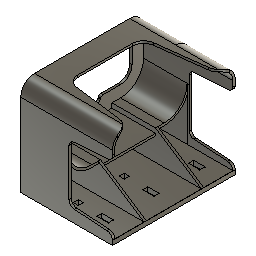
brother_e550w_holder (Autodesk Fusion 360 design; units mm, degrees)
Autodesk Fusion 360 part; units mm, degrees
sketch "Sketch1" plane through (0, 0, 0) normal (1, 0, 0) x (0, 1, 0)
  line L0 (103, 20) -> (103, 42)
  line L1 (93, 52) -> (10, 52)
  line L2 (0, 42) -> (0, 20)
  arc A0 (0, 20) -> (20, 0) centre (20, 20) ccw
  arc A1 (83, 0) -> (103, 20) centre (83, 20) ccw
  arc A2 (10, 52) -> (0, 42) centre (10, 42) ccw
  arc A3 (103, 42) -> (93, 52) centre (93, 42) ccw
  line L3 (51.5, 0) -> (51.5, 52) construction
  line L4 (75.5, 0) -> (75.5, -4)
  line L5 (75.5, -4) -> (27.5, -4)
  line L6 (27.5, -4) -> (27.5, 0)
  line L7 (20, 0) -> (27.5, 0)
  line L8 (75.5, 0) -> (83, 0)
  line L9 (25.5, -6) -> (25.5, -2)
  line L10 (20, -2) -> (25.5, -2)
  arc A4 (-2, 20) -> (20, -2) centre (20, 20) ccw
  line L11 (-2, 42) -> (-2, 20)
  arc A5 (10, 54) -> (-2, 42) centre (10, 42) ccw
  line L12 (93, 54) -> (10, 54)
  arc A6 (105, 42) -> (93, 54) centre (93, 42) ccw
  line L13 (105, 20) -> (105, 42)
  arc A7 (83, -2) -> (105, 20) centre (83, 20) ccw
  line L14 (77.5, -2) -> (83, -2)
  line L15 (77.5, -2) -> (77.5, -6)
  line L16 (77.5, -6) -> (25.5, -6)
  line L17 (133, -6) -> (-25, -6) construction
  line L18 (0, 82) -> (0, -25) construction
  line L19 (-2, 20) -> (-2, -30)
  line L20 (-2, -30) -> (105, -30)
  line L21 (105, -30) -> (105, 20)
  line L22 (0, 20) -> (0, -26)
  line L23 (103, -26) -> (103, 20)
  line L24 (103, -26) -> (0, -26)
  line L25 (25.5, -6) -> (27.5, -6)
  line L26 (27.5, -6) -> (27.5, -26)
  line L27 (27.5, -26) -> (25.5, -26)
  line L28 (25.5, -26) -> (25.5, -6)
  line L29 (75.5, -4) -> (77.5, -4)
  line L30 (77.5, -4) -> (77.5, -26)
  line L31 (77.5, -26) -> (75.5, -26)
  line L32 (75.5, -26) -> (75.5, -4)
  point P0 (103, 0)
  point P1 (0, 52)
  dimension "d1" = 103
  dimension "d2" = 52
  dimension "d3" = 20
  dimension "d4" = 20
  dimension "d5" = 10
  dimension "d6" = 10
  dimension "d7" = 48
  dimension "d8" = 4
  dimension "d56" = 4
  dimension "d57" = 30
  dimension "d58" = 2
  constraint horizontal L7
  constraint vertical L0
  constraint horizontal L1
  constraint vertical L2
  constraint coincident origin L7
  constraint coincident origin L2
  constraint tangent A0 L7
  constraint tangent L2 A0
  constraint coincident P0 L7
  constraint coincident P0 L0
  constraint tangent A1 L7
  constraint tangent L0 A1
  constraint coincident P1 L1
  constraint coincident P1 L2
  constraint tangent L1 A2
  constraint tangent L2 A2
  constraint tangent L0 A3
  constraint tangent L1 A3
  constraint midpoint L1 L3.end
  constraint vertical L4
  constraint horizontal L5
  constraint vertical L6
  constraint symmetric L3 L4 L6
  constraint collinear L7 L8
  constraint coincident L3.start L7
  constraint parallel L6 L9
  constraint parallel L7 L10
  constraint concentric A0 A4
  constraint parallel L2 L11
  constraint concentric A2 A5
  constraint parallel L1 L12
  constraint concentric A3 A6
  constraint parallel L0 L13
  constraint concentric A1 A7
  constraint parallel L8 L14
  constraint parallel L4 L15
  constraint parallel L5 L16
  constraint tangent A7 L14
  constraint tangent L13 A7
  constraint tangent L12 A6
  constraint tangent A5 L12
  constraint tangent A6 L13
  constraint tangent L11 A5
  constraint tangent L10 A4
  constraint tangent A4 L11
  constraint perpendicular L6 L17
  constraint vertical L18
  constraint symmetric L3 L9 L15
  constraint tangent A4 L19
  constraint perpendicular L11 L20
  constraint tangent A7 L21
  constraint coincident L18 L22.end
  constraint tangent A0 L22
  constraint tangent A1 L23
  constraint perpendicular L22 L24
  constraint horizontal L25
  constraint vertical L26
  constraint horizontal L27
  constraint vertical L28
  constraint coincident L24 L26.end
  constraint collinear L6 L26
  constraint horizontal L29
  constraint vertical L30
  constraint horizontal L31
  constraint vertical L32
  constraint coincident L24 L30.end
  constraint collinear L15 L30
  measures "d1" distance of origin P0
  measures "d2" distance of origin P1
  measures "d3" radius of A0
  measures "d4" radius of A1
  measures "d5" radius of A2
  measures "d6" radius of A3
  measures "d7" distance of L4.end L5.end
  measures "d8" distance of L5 L7
  measures "d56" distance of L20 L24
  measures "d57" distance of L7 L20
  measures "d58" distance of L26 L28
extrude "Extrude1" add sketch "Sketch1" along normal blind 40 contours A1 L4 L8 A7 L14 L15 L23 L29 | L0 L1 L2 A2 A3 A4 L11 A5 L12 A6 L13 A7 L22 L23 | A4 A7 L19 L20 L21 L22 L23 L24 L27 L31 | A0 L5 L6 L7 L9 L10 A4 L16 L22 L25 L32 | L15 L16 L29 L30 L32 | L16 L24 L30 L31 L32 | L16 L24 L25 L26 L27 L28
sketch "Sketch8" plane through (0, 0, 0) normal (-1, 0, 0) x (0, -1, 0)
  line L0 (-77.5, -2) -> (-77.5, -26)
  line L1 (-77.5, -26) -> (-103, -26)
  line L2 (-103, -26) -> (-103, 10.8348)
  arc A0 (-103, 10.8348) -> (-83, -2) centre (-83, 20) ccw
  line L3 (-83, -2) -> (-77.5, -2)
  line L4 (-75.5, -26) -> (-75.5, -6)
  line L5 (-75.5, -6) -> (-27.5, -6)
  line L6 (-27.5, -6) -> (-27.5, -26)
  line L7 (-27.5, -26) -> (-75.5, -26)
  line L8 (0, 10.8348) -> (0, -26)
  line L9 (0, -26) -> (-25.5, -26)
  line L10 (-25.5, -26) -> (-25.5, -2)
  line L11 (-25.5, -2) -> (-20, -2)
  arc A1 (-20, -2) -> (0, 10.8348) centre (-20, 20) ccw
  line L12 (-75.5, -4) -> (-75.5, 0)
  line L13 (-75.5, 0) -> (-83, 0)
  arc A2 (-103, 20) -> (-83, 0) centre (-83, 20) ccw
  line L14 (-103, 20) -> (-103, 42)
  arc A3 (-93, 52) -> (-103, 42) centre (-93, 42) ccw
  line L15 (-93, 52) -> (-10, 52)
  arc A4 (0, 42) -> (-10, 52) centre (-10, 42) ccw
  line L16 (0, 42) -> (0, 20)
  arc A5 (-20, 0) -> (0, 20) centre (-20, 20) ccw
  line L17 (-20, 0) -> (-27.5, 0)
  line L18 (-27.5, 0) -> (-27.5, -4)
  line L19 (-27.5, -4) -> (-75.5, -4)
  line L20 (-105, 20) -> (-105, -30)
  line L21 (-105, -30) -> (2, -30)
  line L22 (2, -30) -> (2, 42)
  arc A6 (2, 42) -> (-10, 54) centre (-10, 42) ccw
  line L23 (-10, 54) -> (-93, 54)
  arc A7 (-93, 54) -> (-105, 42) centre (-93, 42) ccw
  line L24 (-105, 42) -> (-105, 20)
  line L25 (-10, 34) -> (-10, 20)
  arc A8 (-20, 10) -> (-10, 20) centre (-20, 20) ccw
  line L26 (-20, 10) -> (-35, 10)
  line L27 (-37.5, 7.5) -> (-37.5, 8.5)
  line L28 (-40, 6) -> (-63, 6)
  line L29 (-65.5, 8.5) -> (-65.5, 7.5)
  line L30 (-68, 10) -> (-83, 10)
  arc A9 (-93, 20) -> (-83, 10) centre (-83, 20) ccw
  line L31 (-93, 20) -> (-93, 34)
  line L32 (-85, 42) -> (-18, 42)
  line L33 (-77.5, -2) -> (-83, -2)
  arc A10 (-105, 20) -> (-83, -2) centre (-83, 20) ccw
  line L34 (-105, 20) -> (-105, 42)
  arc A11 (-93, 54) -> (-105, 42) centre (-93, 42) ccw
  line L35 (-93, 54) -> (-10, 54)
  arc A12 (2, 42) -> (-10, 54) centre (-10, 42) ccw
  line L36 (2, 42) -> (2, 20)
  arc A13 (-20, -2) -> (2, 20) centre (-20, 20) ccw
  line L37 (-20, -2) -> (-25.5, -2)
  line L38 (-25.5, -2) -> (-25.5, -6)
  line L39 (-25.5, -6) -> (-77.5, -6)
  line L40 (-77.5, -6) -> (-77.5, -2)
  arc A14 (-85, 42) -> (-93, 34) centre (-85, 34) ccw
  arc A15 (-10, 34) -> (-18, 42) centre (-18, 34) ccw
  arc A16 (-65.5, 7.5) -> (-68, 10) centre (-68, 7.5) ccw
  arc A17 (-65.5, 8.5) -> (-63, 6) centre (-63, 8.5) ccw
  arc A18 (-40, 6) -> (-37.5, 8.5) centre (-40, 8.5) ccw
  arc A19 (-35, 10) -> (-37.5, 7.5) centre (-35, 7.5) ccw
  dimension "d60" = 2
  dimension "d61" = 8
  dimension "d62" = 2.5
  constraint parallel L16 L25
  constraint concentric A5 A8
  constraint parallel L17 L26
  constraint parallel L18 L27
  constraint parallel L19 L28
  constraint parallel L12 L29
  constraint parallel L13 L30
  constraint concentric A2 A9
  constraint parallel L14 L31
  constraint parallel L15 L32
  constraint tangent A9 L31
  constraint tangent L30 A9
  constraint tangent A8 L26
  constraint tangent L25 A8
  constraint tangent L31 A14
  constraint tangent L32 A14
  constraint tangent L25 A15
  constraint tangent L32 A15
  constraint equal A14 A15
  constraint tangent L29 A16
  constraint tangent L30 A16
  constraint tangent L28 A17
  constraint tangent L29 A17
  constraint equal A16 A17
  constraint tangent L27 A18
  constraint tangent L28 A18
  constraint equal A16 A18
  constraint tangent L26 A19
  constraint tangent L27 A19
  constraint equal A16 A19
  measures "d61" radius of A14
  measures "d62" radius of A16
extrude "Extrude6" add sketch "Sketch8" against normal blind 2 contours L12 L13 A2 L14 A3 L15 A4 L16 A5 L17 L18 L19
sketch "Sketch9" plane through (40, 0, 0) normal (1, 0, 0) x (0, 1, 0)
  line L0 (77.5, -26) -> (77.5, -2)
  line L1 (77.5, -2) -> (83, -2)
  arc A0 (83, -2) -> (103, 10.8348) centre (83, 20) ccw
  line L2 (103, 10.8348) -> (103, -26)
  line L3 (103, -26) -> (77.5, -26)
  line L4 (75.5, -6) -> (75.5, -26)
  line L5 (75.5, -26) -> (27.5, -26)
  line L6 (27.5, -26) -> (27.5, -6)
  line L7 (27.5, -6) -> (75.5, -6)
  line L8 (0, -26) -> (0, 10.8348)
  arc A1 (0, 10.8348) -> (20, -2) centre (20, 20) ccw
  line L9 (20, -2) -> (25.5, -2)
  line L10 (25.5, -2) -> (25.5, -26)
  line L11 (25.5, -26) -> (0, -26)
  line L12 (75.5, 0) -> (75.5, -4)
  line L13 (75.5, -4) -> (27.5, -4)
  line L14 (27.5, -4) -> (27.5, 0)
  line L15 (27.5, 0) -> (20, 0)
  arc A2 (0, 20) -> (20, 0) centre (20, 20) ccw
  line L16 (0, 20) -> (0, 42)
  arc A3 (10, 52) -> (0, 42) centre (10, 42) ccw
  line L17 (10, 52) -> (93, 52)
  arc A4 (103, 42) -> (93, 52) centre (93, 42) ccw
  line L18 (103, 42) -> (103, 20)
  arc A5 (83, 0) -> (103, 20) centre (83, 20) ccw
  line L19 (83, 0) -> (75.5, 0)
  line L20 (105, -30) -> (105, 20)
  line L21 (105, 20) -> (105, 42)
  arc A6 (105, 42) -> (93, 54) centre (93, 42) ccw
  line L22 (93, 54) -> (10, 54)
  arc A7 (10, 54) -> (-2, 42) centre (10, 42) ccw
  line L23 (-2, 42) -> (-2, -30)
  line L24 (-2, -30) -> (105, -30)
  arc A8 (103, 42) -> (93, 52) centre (93, 42) ccw
  line L25 (93, 52) -> (10, 52)
  arc A9 (10, 52) -> (0, 42) centre (10, 42) ccw
  line L26 (0, 42) -> (0, -28)
  line L27 (0, -28) -> (103, -28)
  line L28 (103, -28) -> (103, 20)
  line L29 (103, 20) -> (103, 42)
  line L30 (-2, -30) -> (105, -30)
  line L31 (-2, -30) -> (-2, 42)
  line L32 (10, 54) -> (93, 54)
  line L33 (105, 42) -> (105, -30)
  arc A10 (10, 54) -> (-2, 42) centre (10, 42) ccw
  arc A11 (105, 42) -> (93, 54) centre (93, 42) ccw
  line L34 (0, -28) -> (103, -28)
  line L35 (103, -28) -> (103, -26)
  line L36 (103, -26) -> (0, -26)
  line L37 (0, -26) -> (0, -28)
  dimension "d65" = -2
  dimension "d66" = 12
  constraint coincident L23.end L24.start
  constraint coincident L20.start L24.end
  constraint perpendicular L22 L31
  constraint perpendicular L31 L32
  constraint tangent L31 A10
  constraint tangent L32 A10
  constraint tangent L32 A11
  constraint tangent L33 A11
  constraint equal A10 A11
  constraint horizontal L34
  constraint vertical L35
  constraint horizontal L36
  constraint vertical L37
  constraint coincident L2.end L3.start
  measures "d66" radius of A10
extrude "Extrude7" add sketch "Sketch9" along normal blind 40 contours L3 L5 L11 L26 L27 L28 L34 L35 L36 L37 | L20 L21 A6 L22 A7 L23 L24 L30 L31 L32 L33 A10 A11
sketch "Sketch10" plane through (0, 0, 54) normal (0, 0, 1) x (-1, 0, 0)
  line L0 (0, -93) -> (0, -10)
  line L1 (0, -10) -> (-80, -10)
  line L2 (-80, -10) -> (-80, -93)
  line L3 (-80, -93) -> (-40, -93)
  line L4 (-40, -93) -> (0, -93)
  line L5 (-80, -51.5) -> (0, -51.5) construction
  line L6 (-80, -91.5) -> (-20, -84)
  line L7 (-20, -84) -> (-20, -19)
  line L8 (-20, -19) -> (-80, -11.5)
  dimension "d69" = 60
  dimension "d70" = 80
  dimension "d71" = 65
  constraint midpoint L2 L5.start
  constraint midpoint L0 L5.end
  constraint coincident L2 L6.start
  constraint perpendicular L5 L7
  constraint coincident L2 L8.end
  constraint symmetric L5 L6 L8
  measures "d69" distance of L2 L7
  measures "d70" distance of L6.start L8.end
  measures "d71" distance of L6.end L7.end
extrude "Extrude8" cut sketch "Sketch10" against normal up to surface (2 mm away) contours L2 L6 L7 L8
sketch "Sketch11" plane through (0, 0, -30) normal (0, 0, -1) x (1, 0, 0)
  line L0 (0, 2) -> (0, -105)
  line L1 (0, -105) -> (40, -105)
  line L2 (40, -105) -> (80, -105)
  line L3 (80, -105) -> (80, 2)
  line L4 (80, 2) -> (0, 2)
  line L5 (0, -51.5) -> (80, -51.5) construction
  line L6 (65, -49.25) -> (55, -49.25)
  line L7 (55, -49.25) -> (55, -53.75)
  line L8 (55, -53.75) -> (65, -53.75)
  line L9 (65, -53.75) -> (65, -49.25)
  line L10 (39, -49.25) -> (34.5, -49.25)
  line L11 (34.5, -49.25) -> (34.5, -53.75)
  line L12 (34.5, -53.75) -> (39, -53.75)
  line L13 (39, -53.75) -> (39, -49.25)
  line L14 (39, -93.75) -> (39, -89.25)
  line L15 (55, -89.25) -> (55, -93.75)
  line L16 (65, -89.25) -> (55, -89.25)
  line L17 (34.5, -89.25) -> (34.5, -93.75)
  line L18 (65, -93.75) -> (65, -89.25)
  line L19 (39, -89.25) -> (34.5, -89.25)
  line L20 (34.5, -93.75) -> (39, -93.75)
  line L21 (55, -93.75) -> (65, -93.75)
  line L22 (39, -13.75) -> (39, -9.25)
  line L23 (55, -9.25) -> (55, -13.75)
  line L24 (65, -9.25) -> (55, -9.25)
  line L25 (34.5, -9.25) -> (34.5, -13.75)
  line L26 (65, -13.75) -> (65, -9.25)
  line L27 (39, -9.25) -> (34.5, -9.25)
  line L28 (34.5, -13.75) -> (39, -13.75)
  line L29 (55, -13.75) -> (65, -13.75)
  dimension "d74" = 4.5
  dimension "d76" = 16
  dimension "d77" = 10
  dimension "d78" = 15
  dimension "d81" = 0
  dimension "d82" = 40
  constraint midpoint L0 L5.start
  constraint midpoint L3 L5.end
  constraint horizontal L6
  constraint vertical L7
  constraint horizontal L8
  constraint vertical L9
  constraint horizontal L10
  constraint vertical L11
  constraint horizontal L12
  constraint vertical L13
  constraint collinear L6 L10
  constraint collinear L8 L12
  constraint equal L7 L10
  constraint symmetric L5 L6 L8
  measures "d74" distance of L6.start L8.end
  measures "d76" distance of L7 L13
  measures "d77" distance of L6.start L6.end
  measures "d78" distance of L3 L9
extrude "Extrude9" cut sketch "Sketch11" against normal up to surface (4 mm away) contours L6 L7 L8 L9 | L10 L11 L12 L13 | L14 L17 L19 L20 | L15 L16 L18 L21 | L22 L25 L27 L28 | L23 L24 L26 L29
sketch "Sketch13" plane through (40, 0, 0) normal (1, 0, 0) x (0, 1, 0)
  line L0 (25.5, -26) -> (27.5, -26)
  line L1 (27.5, -26) -> (27.5, -6)
  line L2 (27.5, -6) -> (75.5, -6)
  line L3 (75.5, -6) -> (75.5, -26)
  line L4 (75.5, -26) -> (77.5, -26)
  line L5 (77.5, -26) -> (77.5, -2)
  line L6 (77.5, -2) -> (83, -2)
  arc A0 (83, -2) -> (103, 10.8348) centre (83, 20) ccw
  line L7 (103, 10.8348) -> (103, 20)
  arc A1 (83, 0) -> (103, 20) centre (83, 20) ccw
  line L8 (83, 0) -> (75.5, 0)
  line L9 (75.5, 0) -> (75.5, -4)
  line L10 (75.5, -4) -> (27.5, -4)
  line L11 (27.5, -4) -> (27.5, 0)
  line L12 (27.5, 0) -> (20, 0)
  arc A2 (0, 20) -> (20, 0) centre (20, 20) ccw
  line L13 (0, 20) -> (0, 10.8348)
  arc A3 (0, 10.8348) -> (20, -2) centre (20, 20) ccw
  line L14 (20, -2) -> (25.5, -2)
  line L15 (25.5, -2) -> (25.5, -26)
  line L16 (27.5, 0) -> (25.5, 0)
  line L17 (25.5, 0) -> (25.5, -26)
  line L18 (25.5, -26) -> (27.5, -26)
  line L19 (27.5, -26) -> (27.5, 0)
  line L20 (75.5, 0) -> (77.5, 0)
  line L21 (77.5, 0) -> (77.5, -26)
  line L22 (77.5, -26) -> (75.5, -26)
  line L23 (75.5, -26) -> (75.5, 0)
  constraint horizontal L16
  constraint vertical L17
  constraint horizontal L18
  constraint vertical L19
  constraint coincident L0.start L15.end
  constraint coincident L11.end L12.start
  constraint horizontal L20
  constraint vertical L21
  constraint horizontal L22
  constraint vertical L23
  constraint coincident L4.end L5.start
  constraint coincident L8.end L9.start
extrude "Extrude11" add sketch "Sketch13" along normal up to surface (40 mm away) contours L0 L1 L11 L12 L15 L16 L17 L18 L19 | L3 L4 L5 L8 L9 L20 L21 L22 L23
chamfer "Chamfer2" distance 40 distance2 26 2 edges at (80, 76.5, 0) (80, 26.5, 0) measured on face at (14.6667, 78.6667, 0) measured on face at (14.6667, 24.3333, 0)
fillet "Fillet6" radius 10 4 edges at (80, 91.5, 53) (20, 84, 53) (80, 11.5, 53) (20, 19, 53)
sketch "Sketch14" plane through (0, 105, 0) normal (0, 1, 0) x (-1, 0, 0)
  line L0 (-40, 20) -> (-40, 42)
  line L1 (-40, 42) -> (-80, 42)
  line L2 (-80, 42) -> (-80, -30)
  line L3 (-80, -30) -> (-40, -30)
  line L4 (-40, -30) -> (-40, 20)
  line L5 (-80, 33.5) -> (-42, 31)
  line L6 (-42, 31) -> (-42, -19)
  line L7 (-42, -19) -> (-80, -21.5)
  line L8 (-80, 6) -> (-40, 6) construction
  dimension "d93" = 2
  dimension "d94" = 55
  dimension "d95" = 50
  constraint coincident L2 L5.start
  constraint parallel L0 L6
  constraint coincident L2 L7.end
  constraint midpoint L2 L8.start
  constraint coincident L4 L8.end
  constraint perpendicular L4 L8
  constraint symmetric L5 L7 L8
  measures "d93" distance of L4 L6
  measures "d94" distance of L5.start L7.end
  measures "d95" distance of L5.end L6.end
extrude "Extrude12" cut sketch "Sketch14" against normal up to surface (2 mm away) contours L2 L5 L6 L7
fillet "Fillet7" radius 4 4 edges at (80, 104, -21.5) (42, 104, -19) (42, 104, 31) (80, 104, 33.5)
sketch "Sketch15" plane through (0, -2, 0) normal (0, -1, 0) x (1, 0, 0)
  line L0 (0, 42) -> (0, -30)
  line L1 (0, -30) -> (80, -30)
  line L2 (80, -30) -> (80, 42)
  line L3 (80, 42) -> (0, 42)
  line L4 (80, 6) -> (0, 6) construction
  line L5 (80, 33.5) -> (42, 31)
  line L6 (42, 31) -> (42, -19)
  line L7 (42, -19) -> (80, -21.5)
  dimension "d100" = 55
  dimension "d101" = 50
  dimension "d102" = 42
  constraint midpoint L2 L4.start
  constraint midpoint L0 L4.end
  constraint coincident L2 L5.start
  constraint perpendicular L4 L6
  constraint coincident L2 L7.end
  constraint symmetric L4 L5 L7
  measures "d100" distance of L5.start L7.end
  measures "d101" distance of L5.end L6.end
  measures "d102" distance of L0 L6
extrude "Extrude13" cut sketch "Sketch15" against normal up to surface (2 mm away) contours L2 L5 L6 L7
fillet "Fillet8" radius 5 4 edges at (80, -1, 33.5) (80, -1, -21.5) (42, -1, -19) (42, -1, 31)
equation "d4 = d3"
